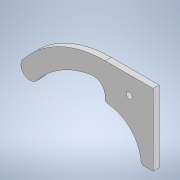
# Autodesk Inventor part: FlexiHook
Saved by Autodesk Inventor 2022 (Build 260153000, 153)
## iProperties
Created: 2022-03-07
Part Number: FlexiHook
Material: Generic
Document SubType Name: Modeling
Designer: tagaz
Density: 1 g/cm^3
Appearance: Default
Author: tagaz
Autodesk Inventor part; units mm, degrees
ref_plane "YZ Plane" through (0, 0, 0) normal (1, 0, 0) x (0, 1, 0)
ref_plane "XZ Plane" through (0, 0, 0) normal (0, 1, 0) x (-1, 0, 0)
ref_plane "XY Plane" through (0, 0, 0) normal (0, 0, 1) x (1, 0, 0)
sketch "Sketch1" plane through (0, 0, 0) normal (0, 0, 1) x (1, 0, 0)
  arc A0 (-1.4591, 69.5225) -> (-81.3996, 30.6287) centre (-1.4591, -32.0775) ccw construction
  arc A1 (-1.4591, 79.0475) -> (-88.894, 36.5074) centre (-1.4591, -32.0775) ccw
  arc A2 (-16.1911, 58.8113) -> (-73.9052, 24.75) centre (-1.4591, -32.0775) ccw
  arc A3 (-88.894, 36.5074) -> (-73.9052, 24.75) centre (-81.3996, 30.6287) ccw
  line L0 (-1.4591, 2.8475) -> (49.3409, 2.8475)
  line L1 (49.3409, 2.8475) -> (49.3409, 79.0475)
  line L2 (49.3409, 79.0475) -> (-1.4591, 79.0475)
  line L3 (-1.4591, 46.2749) -> (-1.4591, 2.8475)
  arc A4 (-1.4591, 46.2749) -> (-16.1911, 58.8113) centre (-14.1591, 46.2749) ccw
  dimension "d5" = 88.9
  dimension "d7" = 50.8
  dimension "d8" = 76.2
  dimension "d9" = 12.7
  dimension "d11" = 50.8
  dimension "d14" = 19.05
  dimension "d15" = 101.6
  constraints: 10 point on circle, 8 end point, 5 centre point, 5 tangent, 2 parallel, 1 horizontal, 1 perpendicular, 1 point on line
  measures "d5" distance of A0.start A0.end
  measures "d7" distance of L2.end L1.end
  measures "d8" distance of L1.end L0.end
  measures "d9" radius of A4
  measures "d11" distance of L0.start L0.end
  measures "d14" radial gap between concentric circles of A2 A1
  measures "d15" radius of A0
extrude "Extrusion1" add sketch "Sketch1" along normal blind 6.35
sketch "Sketch2" plane through (0, 0, 6.35) normal (0, 0, 1) x (1, 0, 0)
  line L0 (-1.4591, 2.8475) -> (49.3409, 2.8475) projected
  circle A0 centre (-1.4591, 2.8475) radius 38.1
  point P0 (0, 0)
  dimension "d16" = 76.2
  constraints: 1 centre point
  measures "d16" diameter of A0
extrude "Extrusion2" cut sketch "Sketch2" against normal blind 6.35
fillet "Fillet1" radius 3.175 2 edges at (-1.4591, 40.9475, 3.175) (36.6409, 2.8475, 3.175)
sketch "Sketch3" plane through (0, 0, 6.35) normal (0, 0, 1) x (1, 0, 0)
  circle A0 centre (23.9409, 59.9975) radius 3.175
  line L0 (49.3409, 79.0475) -> (-1.4591, 79.0475) projected
  line L1 (39.6936, 2.8475) -> (49.3409, 2.8475) projected
  point P0 (0, 0)
  point P1 (23.9409, 79.0475)
  dimension "d20" = 6.35
  dimension "d22" = 19.05
  constraints: 1 centre point, 1 midpoint, 1 vertical alignment
  measures "d20" diameter of A0
  measures "d22" distance from line of L0 A0.centre
extrude "Extrusion3" cut sketch "Sketch3" against normal blind 6.35
sketch "Sketch4" plane through (0, 0, 6.35) normal (0, 0, 1) x (1, 0, 0)
  circle A0 centre (31.075, 15.5475) radius 3.175 construction
  line L0 (49.3409, 79.0475) -> (-1.4591, 79.0475) construction
  arc A1 (36.528, 5.7782) -> (1.4717, 40.8346) centre (-1.4591, 2.8475) ccw construction
  point P0 (0, 0)
  point P1 (23.9409, 79.0475)
  dimension "d25" = 6.35
  dimension "d26" = 63.5
  constraints: 1 centre point, 1 midpoint, 1 tangent
  measures "d25" diameter of A0
  measures "d26" distance from line of L0 A0.centre
body "Solid358"
